Autodesk Inventor part; units mm, degrees
(part 7 of 7)
  line L5147 (-250.4678, -27.1687) -> (-237.9404, -27.1687)
  line L5148 (-242.4092, 5.2493) -> (-242.248, 4.6855)
  line L5149 (-242.248, 4.6855) -> (-242.1115, 4.1155)
  line L5150 (-242.1115, 4.1155) -> (-241.9998, 3.5401)
  line L5151 (-241.9998, 3.5401) -> (-241.9131, 2.9602)
  line L5152 (-241.9131, 2.9602) -> (-241.8115, 2.3363)
  line L5153 (-241.8115, 2.3363) -> (-241.6474, 1.7258)
  line L5154 (-241.6474, 1.7258) -> (-241.5797, 1.5589)
  line L5155 (-241.5797, 1.5589) -> (-241.4919, 1.4025)
  line L5156 (-241.4919, 1.4025) -> (-241.3852, 1.2583)
  line L5157 (-241.3852, 1.2583) -> (-241.2607, 1.1282)
  line L5158 (-241.2607, 1.1282) -> (-241.0368, 0.9696)
  line L5159 (-241.0368, 0.9696) -> (-240.7933, 0.8622)
  line L5160 (-240.7933, 0.8622) -> (-240.5378, 0.8053)
  line L5161 (-240.5378, 0.8053) -> (-240.2781, 0.7985)
  line L5162 (-240.2781, 0.7985) -> (-240.0218, 0.8412)
  line L5163 (-240.0218, 0.8412) -> (-239.7767, 0.9328)
  line L5164 (-239.7767, 0.9328) -> (-239.5504, 1.073)
  line L5165 (-239.5504, 1.073) -> (-239.3506, 1.261)
  line L5166 (-239.3506, 1.261) -> (-239.202, 1.4725)
  line L5167 (-239.202, 1.4725) -> (-239.0876, 1.7026)
  line L5168 (-239.0876, 1.7026) -> (-239.009, 1.9473)
  line L5169 (-239.009, 1.9473) -> (-238.9678, 2.2024)
  line L5170 (-238.9678, 2.2024) -> (-238.948, 2.4129)
  line L5171 (-238.948, 2.4129) -> (-238.9404, 2.6243)
  line L5172 (-238.9404, 2.6243) -> (-238.9639, 3.0579)
  line L5173 (-238.9639, 3.0579) -> (-239.0381, 3.4641)
  line L5174 (-239.0381, 3.4641) -> (-239.1592, 3.8469)
  line L5175 (-239.1592, 3.8469) -> (-239.3271, 4.2063)
  line L5176 (-239.3271, 4.2063) -> (-239.542, 4.5305)
  line L5177 (-239.542, 4.5305) -> (-239.7881, 4.8079)
  line L5178 (-239.7881, 4.8079) -> (-240.0732, 5.0383)
  line L5179 (-240.0732, 5.0383) -> (-240.3935, 5.2219)
  line L5180 (-240.3935, 5.2219) -> (-240.6493, 5.3168)
  line L5181 (-240.6493, 5.3168) -> (-240.9121, 5.3877)
  line L5182 (-240.9121, 5.3877) -> (-241.1803, 5.4343)
  line L5183 (-241.1803, 5.4343) -> (-241.4521, 5.4563)
  line L5184 (-241.4521, 5.4563) -> (-241.9735, 5.473)
  line L5185 (-241.9735, 5.473) -> (-242.4951, 5.4719)
  line L5186 (-242.4951, 5.4719) -> (-242.4092, 5.2493)
  line L5187 (-245.9326, -21.4226) -> (-245.8431, -21.8862)
  line L5188 (-245.8431, -21.8862) -> (-245.668, -22.3199)
  line L5189 (-245.668, -22.3199) -> (-245.4132, -22.7123)
  line L5190 (-245.4132, -22.7123) -> (-245.0849, -23.0515)
  line L5191 (-245.0849, -23.0515) -> (-244.8393, -23.24)
  line L5192 (-244.8393, -23.24) -> (-244.5746, -23.3988)
  line L5193 (-244.5746, -23.3988) -> (-244.2936, -23.5266)
  line L5194 (-244.2936, -23.5266) -> (-243.999, -23.6218)
  line L5195 (-243.999, -23.6218) -> (-243.6251, -23.7112)
  line L5196 (-243.6251, -23.7112) -> (-243.2462, -23.773)
  line L5197 (-243.2462, -23.773) -> (-242.8638, -23.8071)
  line L5198 (-242.8638, -23.8071) -> (-242.4795, -23.8132)
  line L5199 (-242.4795, -23.8132) -> (-242.0932, -23.807)
  line L5200 (-242.0932, -23.807) -> (-241.7089, -23.7729)
  line L5201 (-241.7089, -23.7729) -> (-241.328, -23.7111)
  line L5202 (-241.328, -23.7111) -> (-240.9521, -23.6218)
  line L5203 (-240.9521, -23.6218) -> (-240.6575, -23.5266)
  line L5204 (-240.6575, -23.5266) -> (-240.3765, -23.3988)
  line L5205 (-240.3765, -23.3988) -> (-240.1119, -23.24)
  line L5206 (-240.1119, -23.24) -> (-239.8662, -23.0515)
  line L5207 (-239.8662, -23.0515) -> (-239.667, -22.863)
  line L5208 (-239.667, -22.863) -> (-239.4917, -22.6555)
  line L5209 (-239.4917, -22.6555) -> (-239.3413, -22.4311)
  line L5210 (-239.3413, -22.4311) -> (-239.2169, -22.1922)
  line L5211 (-239.2169, -22.1922) -> (-239.1194, -21.9412)
  line L5212 (-239.1194, -21.9412) -> (-239.0499, -21.6801)
  line L5213 (-239.0499, -21.6801) -> (-239.0094, -21.4115)
  line L5214 (-239.0094, -21.4115) -> (-238.999, -21.1375)
  line L5215 (-238.999, -21.1375) -> (-239.0105, -20.8647)
  line L5216 (-239.0105, -20.8647) -> (-239.0518, -20.5973)
  line L5217 (-239.0518, -20.5973) -> (-239.1221, -20.3377)
  line L5218 (-239.1221, -20.3377) -> (-239.2202, -20.0881)
  line L5219 (-239.2202, -20.0881) -> (-239.3451, -19.8508)
  line L5220 (-239.3451, -19.8508) -> (-239.4957, -19.628)
  line L5221 (-239.4957, -19.628) -> (-239.6711, -19.422)
  line L5222 (-239.6711, -19.422) -> (-239.8701, -19.2351)
  line L5223 (-239.8701, -19.2351) -> (-240.12, -19.0466)
  line L5224 (-240.12, -19.0466) -> (-240.3887, -18.8878)
  line L5225 (-240.3887, -18.8878) -> (-240.6734, -18.7601)
  line L5226 (-240.6734, -18.7601) -> (-240.9717, -18.6648)
  line L5227 (-240.9717, -18.6648) -> (-241.3555, -18.5756)
  line L5228 (-241.3555, -18.5756) -> (-241.7442, -18.5138)
  line L5229 (-241.7442, -18.5138) -> (-242.1362, -18.4797)
  line L5230 (-242.1362, -18.4797) -> (-242.5303, -18.4734)
  line L5231 (-242.5303, -18.4734) -> (-242.9039, -18.4804)
  line L5232 (-242.9039, -18.4804) -> (-243.2756, -18.5148)
  line L5233 (-243.2756, -18.5148) -> (-243.6437, -18.5763)
  line L5234 (-243.6437, -18.5763) -> (-244.0068, -18.6648)
  line L5235 (-244.0068, -18.6648) -> (-244.4879, -18.8454)
  line L5236 (-244.4879, -18.8454) -> (-244.9225, -19.111)
  line L5237 (-244.9225, -19.111) -> (-245.2997, -19.4533)
  line L5238 (-245.2997, -19.4533) -> (-245.6084, -19.864)
  line L5239 (-245.6084, -19.864) -> (-245.784, -20.2299)
  line L5240 (-245.784, -20.2299) -> (-245.8977, -20.6169)
  line L5241 (-245.8977, -20.6169) -> (-245.9478, -21.017)
  line L5242 (-245.9478, -21.017) -> (-245.9326, -21.4226)
  line L5243 (-245.9404, 18.886) -> (-245.8841, 18.5835)
  line L5244 (-245.8841, 18.5835) -> (-245.7846, 18.2941)
  line L5245 (-245.7846, 18.2941) -> (-245.6438, 18.0223)
  line L5246 (-245.6438, 18.0223) -> (-245.4639, 17.7727)
  line L5247 (-245.4639, 17.7727) -> (-245.1573, 17.4565)
  line L5248 (-245.1573, 17.4565) -> (-244.8079, 17.1926)
  line L5249 (-244.8079, 17.1926) -> (-244.4222, 16.9854)
  line L5250 (-244.4222, 16.9854) -> (-244.0068, 16.8391)
  line L5251 (-244.0068, 16.8391) -> (-243.6474, 16.7528)
  line L5252 (-243.6474, 16.7528) -> (-243.2831, 16.6933)
  line L5253 (-243.2831, 16.6933) -> (-242.9155, 16.6608)
  line L5254 (-242.9155, 16.6608) -> (-242.5459, 16.6555)
  line L5255 (-242.5459, 16.6555) -> (-242.1206, 16.6585)
  line L5256 (-242.1206, 16.6585) -> (-241.6967, 16.6883)
  line L5257 (-241.6967, 16.6883) -> (-241.2756, 16.7446)
  line L5258 (-241.2756, 16.7446) -> (-240.8584, 16.8274)
  line L5259 (-240.8584, 16.8274) -> (-240.6035, 16.9037)
  line L5260 (-240.6035, 16.9037) -> (-240.3589, 17.0067)
  line L5261 (-240.3589, 17.0067) -> (-240.1268, 17.1352)
  line L5262 (-240.1268, 17.1352) -> (-239.9092, 17.2883)
  line L5263 (-239.9092, 17.2883) -> (-239.7324, 17.4316)
  line L5264 (-239.7324, 17.4316) -> (-239.5706, 17.5909)
  line L5265 (-239.5706, 17.5909) -> (-239.4247, 17.7648)
  line L5266 (-239.4247, 17.7648) -> (-239.2959, 17.9524)
  line L5267 (-239.2959, 17.9524) -> (-239.1946, 18.1426)
  line L5268 (-239.1946, 18.1426) -> (-239.1142, 18.3419)
  line L5269 (-239.1142, 18.3419) -> (-239.0553, 18.5486)
  line L5270 (-239.0553, 18.5486) -> (-239.0185, 18.761)
  line L5271 (-239.0185, 18.761) -> (-239.003, 19.2065)
  line L5272 (-239.003, 19.2065) -> (-239.0792, 19.6411)
  line L5273 (-239.0792, 19.6411) -> (-239.2433, 20.0506)
  line L5274 (-239.2433, 20.0506) -> (-239.4912, 20.4211)
  line L5275 (-239.4912, 20.4211) -> (-239.7376, 20.6873)
  line L5276 (-239.7376, 20.6873) -> (-240.0164, 20.9166)
  line L5277 (-240.0164, 20.9166) -> (-240.3237, 21.1062)
  line L5278 (-240.3237, 21.1062) -> (-240.6553, 21.2532)
  line L5279 (-240.6553, 21.2532) -> (-240.9991, 21.3628)
  line L5280 (-240.9991, 21.3628) -> (-241.3497, 21.4457)
  line L5281 (-241.3497, 21.4457) -> (-241.7057, 21.5017)
  line L5282 (-241.7057, 21.5017) -> (-242.0654, 21.5305)
  line L5283 (-242.0654, 21.5305) -> (-242.472, 21.5431)
  line L5284 (-242.472, 21.5431) -> (-242.8784, 21.533)
  line L5285 (-242.8784, 21.533) -> (-243.2835, 21.5001)
  line L5286 (-243.2835, 21.5001) -> (-243.6865, 21.4446)
  line L5287 (-243.6865, 21.4446) -> (-243.9998, 21.3762)
  line L5288 (-243.9998, 21.3762) -> (-244.3047, 21.2794)
  line L5289 (-244.3047, 21.2794) -> (-244.5994, 21.1548)
  line L5290 (-244.5994, 21.1548) -> (-244.8818, 21.0032)
  line L5291 (-244.8818, 21.0032) -> (-245.142, 20.8101)
  line L5292 (-245.142, 20.8101) -> (-245.3744, 20.5862)
  line L5293 (-245.3744, 20.5862) -> (-245.5763, 20.3344)
  line L5294 (-245.5763, 20.3344) -> (-245.7451, 20.0579)
  line L5295 (-245.7451, 20.0579) -> (-245.8557, 19.7774)
  line L5296 (-245.8557, 19.7774) -> (-245.9256, 19.4857)
  line L5297 (-245.9256, 19.4857) -> (-245.9541, 19.1871)
  line L5298 (-245.9541, 19.1871) -> (-245.9404, 18.886)
  line L5299 (-246.0029, -34.825) -> (-245.9376, -35.1264)
  line L5300 (-245.9376, -35.1264) -> (-245.8305, -35.414)
  line L5301 (-245.8305, -35.414) -> (-245.6837, -35.6834)
  line L5302 (-245.6837, -35.6834) -> (-245.499, -35.9304)
  line L5303 (-245.499, -35.9304) -> (-245.2399, -36.2006)
  line L5304 (-245.2399, -36.2006) -> (-244.95, -36.435)
  line L5305 (-244.95, -36.435) -> (-244.6327, -36.631)
  line L5306 (-244.6327, -36.631) -> (-244.292, -36.7859)
  line L5307 (-244.292, -36.7859) -> (-243.9405, -36.8975)
  line L5308 (-243.9405, -36.8975) -> (-243.582, -36.9817)
  line L5309 (-243.582, -36.9817) -> (-243.2182, -37.0384)
  line L5310 (-243.2182, -37.0384) -> (-242.8506, -37.0671)
  line L5311 (-242.8506, -37.0671) -> (-242.4469, -37.0799)
  line L5312 (-242.4469, -37.0799) -> (-242.0434, -37.0698)
  line L5313 (-242.0434, -37.0698) -> (-241.6412, -37.0369)
  line L5314 (-241.6412, -37.0369) -> (-241.2412, -36.9812)
  line L5315 (-241.2412, -36.9812) -> (-240.9311, -36.9133)
  line L5316 (-240.9311, -36.9133) -> (-240.6297, -36.8159)
  line L5317 (-240.6297, -36.8159) -> (-240.3392, -36.6899)
  line L5318 (-240.3392, -36.6899) -> (-240.0615, -36.5359)
  line L5319 (-240.0615, -36.5359) -> (-239.7574, -36.3034)
  line L5320 (-239.7574, -36.3034) -> (-239.4955, -36.0275)
  line L5321 (-239.4955, -36.0275) -> (-239.2803, -35.7138)
  line L5322 (-239.2803, -35.7138) -> (-239.1162, -35.3679)
  line L5323 (-239.1162, -35.3679) -> (-239.0496, -35.1295)
  line L5324 (-239.0496, -35.1295) -> (-239.0106, -34.8874)
  line L5325 (-239.0106, -34.8874) -> (-238.9988, -34.6439)
  line L5326 (-238.9988, -34.6439) -> (-239.0139, -34.4013)
  line L5327 (-239.0139, -34.4013) -> (-239.0558, -34.1618)
  line L5328 (-239.0558, -34.1618) -> (-239.1241, -33.9278)
  line L5329 (-239.1241, -33.9278) -> (-239.2185, -33.7015)
  line L5330 (-239.2185, -33.7015) -> (-239.3389, -33.4851)
  line L5331 (-239.3389, -33.4851) -> (-239.5465, -33.2077)
  line L5332 (-239.5465, -33.2077) -> (-239.7887, -32.9621)
  line L5333 (-239.7887, -32.9621) -> (-240.0618, -32.7514)
  line L5334 (-240.0618, -32.7514) -> (-240.3623, -32.5789)
  line L5335 (-240.3623, -32.5789) -> (-240.8315, -32.3896)
  line L5336 (-240.8315, -32.3896) -> (-241.3232, -32.2703)
  line L5337 (-241.3232, -32.2703) -> (-241.924, -32.1911)
  line L5338 (-241.924, -32.1911) -> (-242.5281, -32.1641)
  line L5339 (-242.5281, -32.1641) -> (-243.1324, -32.1892)
  line L5340 (-243.1324, -32.1892) -> (-243.7334, -32.2664)
  line L5341 (-243.7334, -32.2664) -> (-244.0458, -32.3357)
  line L5342 (-244.0458, -32.3357) -> (-244.3498, -32.4335)
  line L5343 (-244.3498, -32.4335) -> (-244.6435, -32.5591)
  line L5344 (-244.6435, -32.5591) -> (-244.9248, -32.7117)
  line L5345 (-244.9248, -32.7117) -> (-245.1874, -32.9059)
  line L5346 (-245.1874, -32.9059) -> (-245.4225, -33.1308)
  line L5347 (-245.4225, -33.1308) -> (-245.6275, -33.3834)
  line L5348 (-245.6275, -33.3834) -> (-245.7998, -33.6609)
  line L5349 (-245.7998, -33.6609) -> (-245.9136, -33.9385)
  line L5350 (-245.9136, -33.9385) -> (-245.986, -34.2282)
  line L5351 (-245.986, -34.2282) -> (-246.016, -34.5252)
  line L5352 (-246.016, -34.5252) -> (-246.0029, -34.825)
  line L5353 (-248.9873, -53.0671) -> (-239.417, -53.0671)
  line L5354 (-239.417, -53.0671) -> (-239.417, -50.3953)
  line L5355 (-239.417, -50.3953) -> (-239.42, -49.9513)
  line L5356 (-239.42, -49.9513) -> (-239.451, -49.5087)
  line L5357 (-239.451, -49.5087) -> (-239.51, -49.069)
  line L5358 (-239.51, -49.069) -> (-239.5967, -48.6336)
  line L5359 (-239.5967, -48.6336) -> (-239.6839, -48.3461)
  line L5360 (-239.6839, -48.3461) -> (-239.7975, -48.0687)
  line L5361 (-239.7975, -48.0687) -> (-239.9367, -47.8033)
  line L5362 (-239.9367, -47.8033) -> (-240.1006, -47.5515)
  line L5363 (-240.1006, -47.5515) -> (-240.2998, -47.325)
  line L5364 (-240.2998, -47.325) -> (-240.6201, -47.0476)
  line L5365 (-240.6201, -47.0476) -> (-240.9912, -46.8015)
  line L5366 (-240.9912, -46.8015) -> (-241.4131, -46.5867)
  line L5367 (-241.4131, -46.5867) -> (-241.7722, -46.446)
  line L5368 (-241.7722, -46.446) -> (-242.1396, -46.3289)
  line L5369 (-242.1396, -46.3289) -> (-242.6727, -46.2139)
  line L5370 (-242.6727, -46.2139) -> (-243.2116, -46.1338)
  line L5371 (-243.2116, -46.1338) -> (-243.7545, -46.0887)
  line L5372 (-243.7545, -46.0887) -> (-244.2998, -46.0789)
  line L5373 (-244.2998, -46.0789) -> (-244.7361, -46.0841)
  line L5374 (-244.7361, -46.0841) -> (-245.1712, -46.1126)
  line L5375 (-245.1712, -46.1126) -> (-245.6042, -46.1643)
  line L5376 (-245.6042, -46.1643) -> (-246.0342, -46.239)
  line L5377 (-246.0342, -46.239) -> (-246.3698, -46.3196)
  line L5378 (-246.3698, -46.3196) -> (-246.6969, -46.4276)
  line L5379 (-246.6969, -46.4276) -> (-247.014, -46.5624)
  line L5380 (-247.014, -46.5624) -> (-247.3193, -46.7234)
  line L5381 (-247.3193, -46.7234) -> (-247.6646, -46.9515)
  line L5382 (-247.6646, -46.9515) -> (-247.9802, -47.2169)
  line L5383 (-247.9802, -47.2169) -> (-248.2632, -47.5168)
  line L5384 (-248.2632, -47.5168) -> (-248.5107, -47.8484)
  line L5385 (-248.5107, -47.8484) -> (-248.6465, -48.0972)
  line L5386 (-248.6465, -48.0972) -> (-248.7554, -48.3579)
  line L5387 (-248.7554, -48.3579) -> (-248.8367, -48.6286)
  line L5388 (-248.8367, -48.6286) -> (-248.8896, -48.907)
  line L5389 (-248.8896, -48.907) -> (-248.9674, -49.6688)
  line L5390 (-248.9674, -49.6688) -> (-248.9873, -50.4343)
  line L5391 (-248.9873, -50.4343) -> (-248.9873, -53.0671)
  line L5392 (-245.9443, 28.5344) -> (-245.8916, 28.1936)
  line L5393 (-245.8916, 28.1936) -> (-245.7937, 27.8681)
  line L5394 (-245.7937, 27.8681) -> (-245.6535, 27.5618)
  line L5395 (-245.6535, 27.5618) -> (-245.4738, 27.2784)
  line L5396 (-245.4738, 27.2784) -> (-245.2574, 27.0219)
  line L5397 (-245.2574, 27.0219) -> (-245.0073, 26.7961)
  line L5398 (-245.0073, 26.7961) -> (-244.7262, 26.605)
  line L5399 (-244.7262, 26.605) -> (-244.417, 26.4524)
  line L5400 (-244.417, 26.4524) -> (-244.1586, 26.3592)
  line L5401 (-244.1586, 26.3592) -> (-243.8938, 26.2882)
  line L5402 (-243.8938, 26.2882) -> (-243.624, 26.2397)
  line L5403 (-243.624, 26.2397) -> (-243.3506, 26.2141)
  line L5404 (-243.3506, 26.2141) -> (-243.3506, 31.2805)
  line L5405 (-243.3506, 31.2805) -> (-243.6597, 31.2481)
  line L5406 (-243.6597, 31.2481) -> (-243.9649, 31.1915)
  line L5407 (-243.9649, 31.1915) -> (-244.2647, 31.1111)
  line L5408 (-244.2647, 31.1111) -> (-244.5576, 31.0071)
  line L5409 (-244.5576, 31.0071) -> (-244.8373, 30.861)
  line L5410 (-244.8373, 30.861) -> (-245.0914, 30.6812)
  line L5411 (-245.0914, 30.6812) -> (-245.3173, 30.4709)
  line L5412 (-245.3173, 30.4709) -> (-245.5127, 30.2335)
  line L5413 (-245.5127, 30.2335) -> (-245.6752, 29.9725)
  line L5414 (-245.6752, 29.9725) -> (-245.8022, 29.6912)
  line L5415 (-245.8022, 29.6912) -> (-245.8914, 29.393)
  line L5416 (-245.8914, 29.393) -> (-245.9404, 29.0813)
  line L5417 (-245.9404, 29.0813) -> (-245.956, 28.8079)
  line L5418 (-245.956, 28.8079) -> (-245.9443, 28.5344)
  line L5419 (-248.6982, -40.7742) -> (-248.6982, -42.3132)
  line L5420 (-248.6982, -42.3132) -> (-250.4678, -42.3132)
  line L5421 (-250.4678, -42.3132) -> (-250.4678, -40.7742)
  line L5422 (-250.4678, -40.7742) -> (-248.6982, -40.7742)
  line L5423 (-248.6982, 36.3977) -> (-248.6982, 34.8625)
  line L5424 (-248.6982, 34.8625) -> (-250.4678, 34.8625)
  line L5425 (-250.4678, 34.8625) -> (-250.4678, 36.3977)
  line L5426 (-250.4678, 36.3977) -> (-248.6982, 36.3977)
  point P0 (0, 0)
  constraints: 10854 end point
extrude "Extrusion2" [suppressed]
